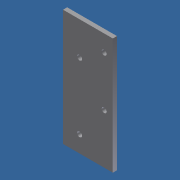
# Autodesk Inventor part: back frame plate
Saved by Autodesk Inventor 2012 (Build 160160000, 160)
## iProperties
Created: 2012-03-16
Part Number: back frame plate
Material: Default
Document SubType Name: Modeling
Designer: Ed
Density: 1 g/cm^3
Author: Ed
Autodesk Inventor part; units mm, degrees
ref_plane "YZ Plane" through (0, 0, 0) normal (1, 0, 0) x (0, 1, 0)
ref_plane "XZ Plane" through (0, 0, 0) normal (0, 1, 0) x (-1, 0, 0)
ref_plane "XY Plane" through (0, 0, 0) normal (0, 0, 1) x (1, 0, 0)
sketch "Sketch1" plane through (0, 0, 0) normal (0, 0, 1) x (1, 0, 0)
  line L0 (0, 0) -> (76.2, 0)
  line L1 (76.2, 0) -> (76.2, 177.8)
  line L2 (76.2, 177.8) -> (0, 177.8)
  line L3 (0, 177.8) -> (0, 0)
  dimension "d0" = 76.2
  dimension "d1" = 177.8
  constraints: 8 end point, 2 parallel, 1 horizontal, 1 perpendicular
  measures "d0" distance of L0.start L0.end
  measures "d1" distance of L2.end L0.start
extrude "Extrusion1" add sketch "Sketch1" along normal blind 6.35
sketch "Sketch2" plane through (0, 0, 6.35) normal (0, 0, 1) x (1, 0, 0)
  line L0 (0, 0) -> (0, 152.4)
  line L1 (76.2, 0) -> (0, 0)
  line L2 (0, 152.4) -> (76.2, 152.4)
  line L3 (0, 177.8) -> (76.2, 177.8) projected
  line L4 (62.9031, 76.2) -> (62.9031, 152.4)
  point P0 (25.4, 25.4)
  point P1 (25.4, 127)
  dimension "d4" = 101.6
  dimension "d5" = 25.4
  dimension "d6" = 25.4
  dimension "d7" = 76.2
  dimension "d17" = 37.5031
  dimension "d18" = 152.4
  constraints: 8 end point, 2 vertical alignment, 1 horizontal alignment, 1 vertical
  measures "d4" distance of point (25.4, 127) point (25.4, 25.4)
  measures "d5" distance from line of L1 point (25.4, 25.4)
  measures "d6" distance from line of L0 point (25.4, 25.4)
  measures "d7" distance of L4.start L4.end
  measures "d17" distance from line of point (25.4, 127) L4
  measures "d18" distance from line of L1 L4.end
hole "Hole1" at (25.4, 25.4, 6.35) at (25.4, 127, 6.35) at (62.9031, 152.4, 6.35) at (62.9031, 76.2, 6.35) direction (0, 0, -1) diameter 7.62 end through all
body "Solid1"
